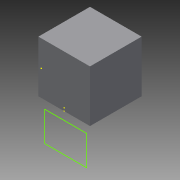
# Autodesk Inventor part: Box01
Saved by Autodesk Inventor 2015 (Build 190159000, 159)
## iProperties
Created: 2016-06-10
Part Number: Box01
Material: Generic
Document SubType Name: Modeling
Designer: Alex
Density: 1 g/cm^3
Appearance: Default
Author: Alex
Autodesk Inventor part; units mm, degrees
ref_plane "YZ Plane" through (0, 0, 0) normal (1, 0, 0) x (0, 1, 0)
ref_plane "XZ Plane" through (0, 0, 0) normal (0, 1, 0) x (-1, 0, 0)
ref_plane "XY Plane" through (0, 0, 0) normal (0, 0, 1) x (1, 0, 0)
sketch "Sketch1" plane through (0, 0, 0) normal (0, 1, 0) x (-1, 0, 0)
  line L0 (25, 25) -> (-25, 25)
  line L1 (-25, 25) -> (-25, -25)
  line L2 (-25, -25) -> (25, -25)
  line L3 (25, -25) -> (25, 25)
  point P0 (0, 0)
  dimension "d0" = 25
  dimension "d1" = 50
  dimension "d2" = 25
  dimension "d3" = 25
  constraints: 8 end point, 2 parallel, 1 horizontal, 1 perpendicular
  measures "d0" distance from line of point (0, 0) L2
  measures "d1" distance between parallel lines of L2 L0
  measures "d2" distance from line of point (0, 0) L3
  measures "d3" distance from line of point (0, 0) L1
extrude "Extrusion1" add sketch "Sketch1" along normal blind 50
sketch "Sketch2" plane through (0, 50, 0) normal (0, 1, 0) x (1, 0, 0)
  line L0 (-22, -22) -> (22, -22)
  line L1 (22, -22) -> (22, 22)
  line L2 (22, 22) -> (-22, 22)
  line L3 (-22, 22) -> (-22, -22)
  point P0 (0, 0)
  dimension "d6" = 22
  dimension "d7" = 22
  dimension "d8" = 22
  dimension "d9" = 22
  constraints: 8 end point, 2 parallel, 1 horizontal, 1 perpendicular
  measures "d6" distance from line of point (0, 0) L3
  measures "d7" distance from line of point (0, 0) L1
  measures "d8" distance from line of point (0, 0) L2
  measures "d9" distance from line of point (0, 0) L0
extrude "Extrusion2" cut sketch "Sketch2" against normal blind 47
sketch "Sketch3" plane through (0, 3, 0) normal (0, 1, 0) x (1, 0, 0)
  circle A0 centre (0, 0) radius 5
  dimension "d12" = 10
  constraints: 1 centre point, 1 coincident
  measures "d12" diameter of A0
extrude "Extrusion3" add sketch "Sketch3" along normal blind 40
sketch "Sketch4" plane through (0, 50, 0) normal (0, 1, 0) x (1, 0, 0)
  line L0 (-22, 22) -> (22, 22)
  line L1 (22, 22) -> (22, 25)
  line L2 (22, 25) -> (-22, 25)
  line L3 (-22, 25) -> (-22, 22)
  line L4 (25, -25) -> (25, 25) projected
  point P0 (0, 0)
  dimension "d15" = 3
  dimension "d16" = 25
  constraints: 8 end point, 2 parallel, 1 horizontal, 1 perpendicular
  measures "d15" distance between parallel lines of L4 L1
  measures "d16" distance from line of point (0, 0) L2
extrude "Extrusion4" cut sketch "Sketch4" against normal blind 3
sketch "Sketch5" plane through (-22, 3, -22) normal (0, 0, 1) x (1, 0, 0)
  point P0 (22, -3)
sketch "Sketch6" plane through (25, 0, -25) normal (0, 0, -1) x (-1, 0, 0)
  line L0 (3, 47) -> (47, 47) projected
  circle A0 centre (25, 47) radius 2
  point P0 (25, 0)
  dimension "d19" = 4
  constraints: 1 centre point, 1 midpoint
  measures "d19" diameter of A0
extrude "Extrusion5" cut sketch "Sketch6" against normal blind 3
sketch "Sketch7" plane through (-22, 50, 22) normal (1, 0, 0) x (0, 0, -1)
  point P0 (22, -50)
sketch "Sketch8" plane through (25, 0, -25) normal (0, 0, -1) x (-1, 0, 0)
  line L0 (47, 50) -> (47, 47) projected
  circle A0 centre (47, 48.5) radius 0.75
  line L1 (3, 50) -> (47, 50) projected
  line L2 (3, 47) -> (3, 50) projected
  circle A1 centre (3, 48.5) radius 0.75
  point P0 (25, 0)
  dimension "d22" = 1.5
  dimension "d23" = 1.5
  dimension "d24" = 1.5
  constraints: 2 centre point, 2 midpoint
  measures "d22" distance from line of L1 A0.centre
  measures "d23" diameter of A0
  measures "d24" diameter of A1
extrude "Extrusion6" cut sketch "Sketch8" against normal blind 48.5 contours A0 L0 | L0 A0
sketch "Sketch9" plane through (25, 0, -25) normal (0, 0, -1) x (-1, 0, 0)
  point P0 (25, 0)
sketch "Sketch10" plane through (25, 0, -25) normal (0, 0, -1) x (-1, 0, 0)
  line L0 (3, 50) -> (3, 3) projected
  circle A0 centre (3, 48.5) radius 0.75
  line L1 (3, 50) -> (47, 50) projected
  point P0 (25, 0)
  dimension "d27" = 1.5
  dimension "d28" = 1.5
  constraints: 1 centre point, 1 point on line
  measures "d27" distance from line of L1 A0.centre
  measures "d28" diameter of A0
extrude "Extrusion7" cut sketch "Sketch10" against normal blind 48.5
sketch "Sketch11" plane through (22, 50, 22) normal (0, 0, -1) x (-1, 0, 0)
  line L0 (44, -0.75) -> (0, -0.75)
  line L1 (0, -0.75) -> (0, -2.25)
  line L2 (0, -2.25) -> (44, -2.25)
  line L3 (44, -2.25) -> (44, -0.75)
  point P0 (22, -50)
  constraints: 8 end point, 2 parallel, 1 horizontal, 1 perpendicular
extrude "Extrusion8" cut sketch "Sketch11" against normal blind 1.5
sketch "Sketch12" plane through (0, 3, 0) normal (0, 1, 0) x (1, 0, 0)
  line L0 (-21.9343, 35.7574) -> (18.5832, 35.7574)
  line L1 (18.5832, 35.7574) -> (18.5832, 64.5461)
  line L2 (18.5832, 64.5461) -> (-21.9343, 64.5461)
  line L3 (-21.9343, 64.5461) -> (-21.9343, 35.7574)
  point P0 (0, 0)
  constraints: 8 end point, 2 parallel, 1 horizontal, 1 perpendicular
body "Solid1"
